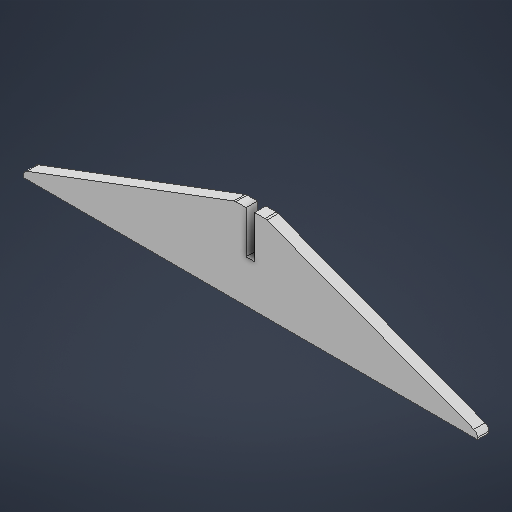
# Autodesk Inventor part: LegLessMaterial
Saved by Autodesk Inventor 2026 (Build 300175000, 175)
## iProperties
Created: 2025-03-30
Part Number: LegLessMaterial
Material: Všeobecné
Document SubType Name: Modeling
Designer: 42060
Density: 1 g/cm^3
Appearance: Výchozí
Author: 42060
Autodesk Inventor part; units mm, degrees
ref_plane "YZ Plane" through (0, 0, 0) normal (1, 0, 0) x (0, 1, 0)
ref_plane "XZ Plane" through (0, 0, 0) normal (0, 1, 0) x (-1, 0, 0)
ref_plane "XY Plane" through (0, 0, 0) normal (0, 0, 1) x (1, 0, 0)
sketch "Náčrt1" plane through (0, 0, 0) normal (0, 0, 1) x (1, 0, 0)
  line L0 (0, 15) -> (-1.5, 15)
  line L1 (-1.5, 15) -> (-1.5, 30)
  line L2 (-1.5, 30) -> (-5.1366, 30)
  line L3 (-5.8402, 29.8721) -> (-78.7036, 2.4872)
  line L4 (-80, 0.6151) -> (-80, 0)
  line L5 (-80, 0) -> (0, 0)
  arc A0 (-78.7036, 2.4872) -> (-80, 0.6151) centre (-78, 0.6151) ccw
  arc A1 (-5.1366, 30) -> (-5.8402, 29.8721) centre (-5.1366, 28) ccw
  line L6 (0, 15) -> (0, 0)
  line L7 (0, 15) -> (1.5, 15)
  line L8 (1.5, 15) -> (1.5, 30)
  line L9 (1.5, 30) -> (5.1366, 30)
  line L10 (5.8402, 29.8721) -> (78.7036, 2.4872)
  line L11 (80, 0.6151) -> (80, 0)
  line L12 (80, 0) -> (0, 0)
  arc A2 (80, 0.6151) -> (78.7036, 2.4872) centre (78, 0.6151) ccw
  arc A3 (5.8402, 29.8721) -> (5.1366, 30) centre (5.1366, 28) ccw
  point P0 (-5.5, 30)
  point P1 (-80, 2)
  point P2 (5.5, 30)
  point P3 (80, 2)
  dimension "d1" = 15
  dimension "d5" = 4
  dimension "d7" = 2
  dimension "d9" = 2
  dimension "d12" = 15
  dimension "d13" = 1.5
  dimension "d14" = 80
  constraints: 26 end point, 11 symmetric about line, 8 point on circle, 8 point on line, 4 centre point, 4 tangent, 2 perpendicular, 2 vertical, 1 equal radius, 1 horizontal, 1 parallel, 2 other
  measures "d1" distance between parallel lines of L5 L0
  measures "d5" distance of L1.end point (-5.5, 30)
  measures "d7" distance of point (-80, 2) L4.end
  measures "d9" radius of A0
  measures "d12" distance of L0.end L1.end
  measures "d13" distance of L0.start L0.end
  measures "d14" distance of L5.end L4.end
extrude "Vysunutí1" add sketch "Náčrt1" along normal mid plane 4
equation "\"d10\" = d4"
equation "\"d4\" = 4"
